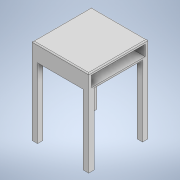
# Autodesk Inventor part: Base_carga
Saved by Autodesk Inventor 2021 (Build 250183000, 183)
## iProperties
Created: 2021-02-07
Part Number: Base_carga
Material: Genérico
Document SubType Name: Modeling
Designer: rotje
Density: 1 g/cm^3
Appearance: Valor por defecto
Author: rotje
Autodesk Inventor part; units mm, degrees
ref_plane "YZ Plane" through (0, 0, 0) normal (1, 0, 0) x (0, 1, 0)
ref_plane "XZ Plane" through (0, 0, 0) normal (0, 1, 0) x (-1, 0, 0)
ref_plane "XY Plane" through (0, 0, 0) normal (0, 0, 1) x (1, 0, 0)
sketch "Boceto1" plane through (0, 0, 0) normal (0, 1, 0) x (-1, 0, 0)
  line L0 (0, 0) -> (0, -55)
  line L1 (0, -55) -> (0, 55)
  line L2 (0, 55) -> (105, 55)
  line L3 (105, 55) -> (105, -55)
  line L4 (105, -55) -> (0, -55)
  dimension "d0" = 55
  dimension "d1" = 110
  dimension "d2" = 105
  dimension "d3" = 110
  constraints: 10 end point, 2 vertical, 1 horizontal, 1 point on line
  measures "d0" distance of L0.start L0.end
  measures "d1" distance of L0.end L1.end
  measures "d2" distance of L1.end L2.end
  measures "d3" distance of L2.end L3.end
extrude "Extrusión1" add sketch "Boceto1" along normal blind 30
sketch "Boceto2" plane through (0, 0, 55) normal (1, 0, 0) x (0, 0, -1)
  line L0 (0, 0) -> (0, 30) projected
  line L1 (0, 0) -> (0, 5)
  line L2 (0, 5) -> (110, 5)
  line L3 (110, 0) -> (110, 30) projected
  line L4 (110, 30) -> (0, 30) projected
  line L5 (0, 30) -> (0, 25)
  line L6 (0, 25) -> (110, 25)
  line L7 (0, 30) -> (5, 30)
  line L8 (5, 30) -> (5, 0)
  line L9 (110, 0) -> (0, 0) projected
  line L10 (110, 30) -> (105, 30)
  line L11 (105, 30) -> (105, 0)
  point P0 (55, 0)
  point P1 (105, 5)
  point P2 (105, 25)
  point P3 (5, 25)
  point P4 (5, 5)
  dimension "d6" = 5
  dimension "d7" = 5
  dimension "d9" = 110
  dimension "d10" = 5
  dimension "d11" = 5
  constraints: 16 end point, 7 point on line, 3 perpendicular
  measures "d6" distance of L0.start L1.end
  measures "d7" distance of L0.end L5.end
  measures "d9" distance of L5.end L6.end
  measures "d10" distance of L0.end L7.end
  measures "d11" distance of L3.end L10.end
extrude "Extrusión2" cut sketch "Boceto2" against normal blind 100 contours L8 L6 L11 L2
sketch "Boceto3" plane through (0, 0, 0) normal (0, -1, 0) x (1, 0, 0)
  line L0 (0, 55.0451) -> (0, 45.0451)
  line L1 (0, -50) -> (0, 50) projected
  line L2 (0, 45.0451) -> (-10, 45.0451)
  line L3 (-105, 55) -> (0, 55) projected
  line L4 (0, 55) -> (-10, 55)
  line L5 (-10, 45.0451) -> (-10, 55)
  line L6 (0, 0) -> (-105, 0)
  line L7 (-105, -55) -> (-105, 55) projected
  line L8 (-105, 55) -> (-105, 45)
  line L9 (-105, 45) -> (-95, 45)
  line L10 (-95, 45) -> (-95, 55)
  line L11 (-105, 55) -> (-95, 55)
  line L12 (0, -55.0451) -> (0, -45.0451)
  line L13 (0, -45.0451) -> (-10, -45.0451)
  line L14 (-105, -55) -> (0, -55)
  line L15 (-10, -45.0451) -> (-10, -55)
  line L16 (-105, 55) -> (-105, -55)
  line L17 (-105, -45) -> (-95, -45)
  line L18 (-95, -45) -> (-95, -55)
  dimension "d14" = 10
  dimension "d15" = 10
  dimension "d16" = 10
  dimension "d17" = 10
  constraints: 32 end point, 10 symmetric about line, 7 point on line, 3 perpendicular, 1 collinear, 1 midpoint, 1 vertical
  measures "d14" distance of L0.start L0.end
  measures "d15" distance of L0.end L2.end
  measures "d16" distance of L3.start L8.end
  measures "d17" distance of L8.end L9.end
extrude "Extrusión3" add sketch "Boceto3" along normal blind 130 contours L0 L2 L5 L3 | L10 L9 L7 L3 | L1 L12 L14 L15 L13 | L17 L18 L14 L7
fillet "Empalme1" radius 2 5 edges at (-52.5, 30, 55) (-52.5, 30, -55) (-105, 30, 0) (0, 30, 0) (0, 0, 0)
